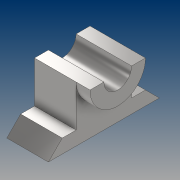
# Autodesk Inventor part: 1
Saved by Autodesk Inventor 2020.2 (Build 242310000, 310)
## iProperties
Created: 2020-09-17
Part Number: 1
Material: 鋼、碳鋼
Document SubType Name: Modeling
Designer: user
Density: 7.85 g/cm^3
Appearance: 半拋光
Mass: 447.45 g
Surface Area: 118.193 cm^2
Volume: 57 cm^3
Author: user
Autodesk Inventor part; units mm, degrees
ref_plane "YZ Plane" through (0, 0, 0) normal (1, 0, 0) x (0, 1, 0)
ref_plane "XZ Plane" through (0, 0, 0) normal (0, 1, 0) x (-1, 0, 0)
ref_plane "XY Plane" through (0, 0, 0) normal (0, 0, 1) x (1, 0, 0)
sketch "草圖1" plane through (0, 0, 0) normal (0, 0, 1) x (1, 0, 0)
  line L0 (0, 0) -> (80, 0)
  line L1 (60, 10) -> (60, 40)
  line L2 (20, 40) -> (20, 10)
  line L3 (20, 10) -> (10, 10)
  line L4 (10, 10) -> (0, 0)
  line L5 (60, 10) -> (70, 10)
  line L6 (70, 10) -> (80, 0)
  arc A0 (20, 40) -> (60, 40) centre (40, 40) ccw
  arc A1 (30, 40) -> (50, 40) centre (40, 40) ccw
  line L7 (60, 40) -> (50, 40)
  line L8 (30, 40) -> (20, 40)
  dimension "d0" = 80
  dimension "d1" = 45
  dimension "d2" = 10
  dimension "d4" = 40
  dimension "d6" = 30
  dimension "d14" = 40
  dimension "d15" = 10
  dimension "d16" = 20
  constraints: 18 end point, 5 perpendicular, 4 point on circle, 2 centre point, 2 equal length, 2 horizontal, 1 coincident, 1 horizontal alignment
  measures "d0" distance of L0.start L0.end
  measures "d1" angle of L0 L4
  measures "d2" distance of L2.end L3.end
  measures "d4" distance of L1.end L2.start
  measures "d6" distance of L1.start L1.end
  measures "d14" distance between parallel lines of L8 L0
  measures "d15" radius of A1
  measures "d16" radius of A0
extrude "擠出1" add sketch "草圖1" along normal blind 30
extrude "擠出2" add sketch "草圖1" along normal blind 40 contours L8 A1 L7 A0
